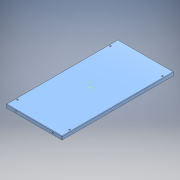
# Autodesk Inventor part: 垃圾桶正版
Saved by Autodesk Inventor 2017 (Build 210142000, 142)
## iProperties
Part Number: 垃圾桶正版
Material: 常规
Document SubType Name: Modeling
Designer: PANDA
Density: 1 g/cm^3
Appearance: 默认
Mass: 3592.32 g
Surface Area: 3957.98 cm^2
Volume: 3592.32 cm^3
Author: PANDA
Autodesk Inventor part; units mm, degrees
ref_plane "YZ Plane" through (0, 0, 0) normal (1, 0, 0) x (0, 1, 0)
ref_plane "XZ Plane" through (0, 0, 0) normal (0, 1, 0) x (-1, 0, 0)
ref_plane "XY Plane" through (0, 0, 0) normal (0, 0, 1) x (1, 0, 0)
sketch "草图1" plane through (0, 0, 0) normal (1, 0, 0) x (0, 1, 0)
  point P0 (0, 0)
sketch "草图2" plane through (0, 0, 0) normal (0, 0, 1) x (1, 0, 0)
  line L0 (-150, -300) -> (150, -300)
  line L1 (150, -300) -> (150, 300)
  line L2 (150, 300) -> (-150, 300)
  line L3 (-150, 300) -> (-150, -300)
  point P0 (0, 0)
  dimension "d0" = 300
  dimension "d1" = 600
  constraints: 8 end point, 2 parallel, 1 horizontal, 1 perpendicular
  measures "d0" distance of L2.end L1.end
  measures "d1" distance of L1.end L0.end
extrude "拉伸1" add sketch "草图2" along normal blind 20
sketch "草图3" plane through (0, 0, 20) normal (0, 0, 1) x (1, 0, 0)
  circle A0 centre (-140, 250) radius 2
  point P0 (0, 0)
  dimension "d4" = 4
  constraints: 1 centre point
  measures "d4" diameter of A0
extrude "拉伸2" cut sketch "草图3" against normal through all
sketch "草图4" plane through (0, 0, 20) normal (0, 0, 1) x (1, 0, 0)
  circle A0 centre (-110, 250) radius 2
  point P0 (0, 0)
  dimension "d7" = 4
  constraints: 1 centre point
  measures "d7" diameter of A0
extrude "拉伸3" cut sketch "草图4" against normal up to next
sketch "草图5" plane through (0, 0, 20) normal (0, 0, 1) x (1, 0, 0)
  circle A0 centre (140, 250) radius 2
  point P0 (0, 0)
  dimension "d10" = 4
  constraints: 1 centre point
  measures "d10" diameter of A0
extrude "拉伸4" cut sketch "草图5" against normal up to next
sketch "草图6" plane through (0, 0, 20) normal (0, 0, 1) x (1, 0, 0)
  circle A0 centre (110, 250) radius 2
  point P0 (0, 0)
  dimension "d13" = 4
  constraints: 1 centre point
  measures "d13" diameter of A0
extrude "拉伸5" cut sketch "草图6" against normal through all
sketch "草图7" plane through (0, 0, 20) normal (0, 0, 1) x (1, 0, 0)
  circle A0 centre (140, -250) radius 2
  point P0 (0, 0)
  dimension "d16" = 4
  constraints: 1 centre point
  measures "d16" diameter of A0
extrude "拉伸6" cut sketch "草图7" against normal through all
sketch "草图9" plane through (0, 0, 20) normal (0, 0, 1) x (1, 0, 0)
  circle A0 centre (-140, -250) radius 2
  point P0 (0, 0)
  dimension "d22" = 4
  constraints: 1 centre point
  measures "d22" diameter of A0
extrude "拉伸8" cut sketch "草图9" against normal through all
sketch "草图11" plane through (-150, -300, 0) normal (0, -1, 0) x (1, 0, 0)
  circle A0 centre (25, 10) radius 2
  point P0 (150, 0)
  dimension "d28" = 4
  constraints: 1 centre point
  measures "d28" diameter of A0
extrude "拉伸10" cut sketch "草图11" against normal blind 20
sketch "草图12" plane through (-150, -300, 0) normal (0, -1, 0) x (1, 0, 0)
  circle A0 centre (275, 10) radius 2
  point P0 (150, 0)
  dimension "d31" = 4
  constraints: 1 centre point
  measures "d31" diameter of A0
extrude "拉伸11" cut sketch "草图12" against normal blind 20
sketch "草图13" plane through (-150, -300, 0) normal (0, -1, 0) x (1, 0, 0)
  circle A0 centre (275, 10) radius 2 projected
  circle A1 centre (275, 10) radius 2
  point P0 (150, 0)
  dimension "d34" = 4
  constraints: 1 centre point, 1 coincident
  measures "d34" diameter of A1
extrude "拉伸12" cut sketch "草图13" against normal blind 40
sketch "草图14" plane through (-150, -300, 0) normal (0, -1, 0) x (1, 0, 0)
  circle A0 centre (25, 10) radius 2 projected
  circle A1 centre (25, 10) radius 2
  point P0 (150, 0)
  dimension "d37" = 4
  constraints: 1 centre point, 1 coincident
  measures "d37" diameter of A1
extrude "拉伸13" cut sketch "草图14" against normal blind 40
sketch "草图15" plane through (-150, -300, 0) normal (0, -1, 0) x (1, 0, 0)
  circle A0 centre (25, 10) radius 2 projected
  circle A1 centre (25, 10) radius 2
  point P0 (150, 0)
  dimension "d40" = 4
  constraints: 1 centre point, 1 coincident
  measures "d40" diameter of A1
extrude "拉伸14" add sketch "草图15" against normal blind 600
sketch "草图16" plane through (-150, -300, 0) normal (0, -1, 0) x (1, 0, 0)
  circle A0 centre (275, 10) radius 2 projected
  circle A1 centre (275, 10) radius 2
  point P0 (150, 0)
  dimension "d43" = 4
  constraints: 1 centre point, 1 coincident
  measures "d43" diameter of A1
extrude "拉伸15" add sketch "草图16" against normal blind 600
sketch "草图17" plane through (-150, -300, 0) normal (0, -1, 0) x (1, 0, 0)
  circle A0 centre (50, 10) radius 2
  point P0 (150, 0)
  dimension "d46" = 4
  constraints: 1 centre point
  measures "d46" diameter of A0
extrude "拉伸16" cut sketch "草图17" against normal blind 40
sketch "草图18" plane through (-150, -300, 0) normal (0, -1, 0) x (1, 0, 0)
  circle A0 centre (250, 10) radius 2
  point P0 (150, 0)
  dimension "d49" = 4
  constraints: 1 centre point
  measures "d49" diameter of A0
extrude "拉伸17" cut sketch "草图18" against normal blind 40
sketch "草图19" plane through (0, 0, 20) normal (0, 0, 1) x (1, 0, 0)
  circle A0 centre (110, 250) radius 3
  point P0 (0, 0)
  dimension "d52" = 6
  constraints: 1 centre point
  measures "d52" diameter of A0
extrude "拉伸18" cut sketch "草图19" against normal through all
sketch "草图20" plane through (0, 0, 20) normal (0, 0, 1) x (1, 0, 0)
  circle A0 centre (-110, 250) radius 2 projected
  circle A1 centre (-110, 250) radius 3
  point P0 (0, 0)
  dimension "d55" = 6
  constraints: 1 centre point, 1 coincident
  measures "d55" diameter of A1
extrude "拉伸19" cut sketch "草图20" against normal through all
sketch "草图21" plane through (0, 0, 20) normal (0, 0, 1) x (1, 0, 0)
  point P0 (0, 0)
sketch "草图24" plane through (0, 0, 20) normal (0, 0, 1) x (1, 0, 0)
  circle A0 centre (-109.8054, 249.5578) radius 2
  point P0 (0, 0)
  dimension "d64" = 4
  constraints: 1 centre point
  measures "d64" diameter of A0
extrude "拉伸22" add sketch "草图24" against normal blind 20
sketch "草图25" plane through (-109.8054, 249.5578, 20) normal (0, 0, 1) x (1, 0, 0)
  point P0 (109.8054, -249.5578)
sketch "草图26" plane through (0, 0, 20) normal (0, 0, 1) x (1, 0, 0)
  circle A0 centre (-110, 250) radius 2
  point P0 (0, 0)
  dimension "d67" = 4
  constraints: 1 centre point
  measures "d67" diameter of A0
extrude "拉伸23" cut sketch "草图26" against normal blind 20
sketch "草图27" plane through (0, 0, 20) normal (0, 0, 1) x (1, 0, 0)
  circle A0 centre (-110, 250) radius 2
  point P0 (0, 0)
  dimension "d70" = 4
  constraints: 1 centre point
  measures "d70" diameter of A0
extrude "拉伸24" add sketch "草图27" against normal blind 20
sketch "草图28" plane through (0, 0, 20) normal (0, 0, 1) x (1, 0, 0)
  arc A0 (-111.7199, 248.9793) -> (-108.0855, 250.5785) centre (-109.8054, 249.5578) ccw projected
  circle A1 centre (-111.7199, 248.9793) radius 12.6213
  point P0 (0, 0)
  constraints: 1 centre point, 1 other
extrude "拉伸25" add sketch "草图28" against normal blind 20
sketch "草图29" plane through (0, 0, 20) normal (0, 0, 1) x (1, 0, 0)
  circle A0 centre (110, 250) radius 3 projected
  circle A1 centre (110, 250) radius 2
  point P0 (0, 0)
  dimension "d75" = 4
  constraints: 1 centre point, 1 coincident
  measures "d75" diameter of A1
extrude "拉伸26" add sketch "草图29" against normal blind 20
sketch "草图30" plane through (0, 0, 20) normal (0, 0, 1) x (1, 0, 0)
  circle A0 centre (88.039, 258.3731) radius 35.0217
  point P0 (0, 0)
  constraints: 1 centre point
extrude "拉伸27" add sketch "草图30" against normal blind 20
fillet "圆角1" radius 2 2 edges at (-102, -260, 10) (98, -260, 10)
fillet "圆角1" radius 2 22 edges at (-150, 0, 20) (0, -300, 20) (150, 0, 20) (0, 300, 20) (-142, -250, 20) (138, -250, 20) (-142, 250, 20) (138, 250, 20) (-150, 300, 10) (-150, -300, 10) (-150, 0, 0) (150, 300, 10) (0, 300, 0) (0, -300, 0) (150, -300, 10) (-102, -300, 10) (98, -300, 10) (150, 0, 0) (-142, -250, 0) (138, -250, 0) (-142, 250, 0) (138, 250, 0)
